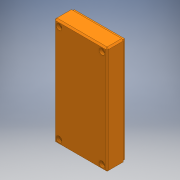
# Autodesk Inventor part: mangOH bottom
Saved by Autodesk Inventor 2017.3 (Build 213256000, 256)
## iProperties
Created: 2018-01-31
Part Number: mangOH bottom
Material: Generic
Document SubType Name: Modeling
Designer: michiel
Density: 1 g/cm^3
Appearance: Orange
Author: michiel
Autodesk Inventor part; units mm, degrees
ref_plane "YZ Plane" through (0, 0, 0) normal (1, 0, 0) x (0, 1, 0)
ref_plane "XZ Plane" through (0, 0, 0) normal (0, 1, 0) x (-1, 0, 0)
ref_plane "XY Plane" through (0, 0, 0) normal (0, 0, 1) x (1, 0, 0)
sketch "Sketch1" plane through (0, 0, 0) normal (0, 1, 0) x (-1, 0, 0)
  line L0 (0, 0) -> (73, 0)
  line L1 (73, 0) -> (73, -148)
  line L2 (73, -148) -> (0, -148)
  line L3 (0, -148) -> (0, 0)
  dimension "d0" = 73
  dimension "d1" = 148
  constraints: 8 end point, 2 parallel, 1 horizontal, 1 perpendicular
  measures "d0" distance of L1.end L2.end
  measures "d1" distance of L0.end L1.end
extrude "Extrusion1" add sketch "Sketch1" against normal blind 4
sketch "Sketch2" plane through (0, 0, 0) normal (0, 1, 0) x (1, 0, 0)
  line L0 (-73, 148) -> (0, 148) projected
  line L1 (0, 148) -> (0, 0) projected
  line L2 (0, 148) -> (0, 0)
  line L3 (0, 0) -> (-73, 0) projected
  line L4 (0, 0) -> (-73, 0)
  line L5 (-73, 0) -> (-73, 148)
  line L6 (0, 148) -> (0, 144) construction
  line L7 (0, 148) -> (0, 0) construction
  line L8 (0, 144) -> (-4, 144) construction
  line L9 (-4, 144) -> (-69, 144)
  line L10 (-69, 144) -> (-69, 4)
  line L11 (-69, 4) -> (-4, 4)
  line L12 (-4, 4) -> (-4, 144)
  dimension "d4" = 4
  dimension "d5" = 4
  dimension "d6" = 90
  dimension "d7" = 65
  dimension "d8" = 140
  constraints: 18 end point, 3 perpendicular, 2 collinear, 2 horizontal, 1 point on line, 1 vertical
  measures "d4" distance of L0.end L6.end
  measures "d5" distance of L6.end L8.end
  measures "d6" angle of L6 L8
  measures "d7" distance of L8.end L9.end
  measures "d8" distance of L9.end L10.end
extrude "Extrusion2" add sketch "Sketch2" along normal blind 22
sketch "Sketch3" plane through (0, 22, 0) normal (0, 1, 0) x (1, 0, 0)
  line L0 (-4, 4) -> (-69, 4)
  line L1 (-4, 4) -> (-2.1, 4) construction
  line L2 (-2.1, 4) -> (-2.1, 2.1) construction
  line L3 (-2.1, 2.1) -> (-71.1, 2.1)
  line L4 (-73, 148) -> (-73, 0) projected
  line L5 (-71.1, 2.1) -> (-71.1, 146.1)
  line L6 (-71.1, 146.1) -> (-2.1, 146.1)
  line L7 (-2.1, 146.1) -> (-2.1, 2.1)
  line L8 (-73, 0) -> (0, 0) projected
  line L9 (0, 148) -> (-73, 148) projected
  line L10 (-73, 0) -> (-73, 148)
  line L11 (-73, 148) -> (0, 148)
  line L12 (0, 148) -> (0, 0)
  point P0 (-4, 144)
  point P1 (-69, 144)
  dimension "d11" = 1.9
  dimension "d12" = 1.9
  dimension "d13" = 69
  dimension "d14" = 144
  dimension "d15" = 69
  constraints: 20 end point, 5 perpendicular, 2 vertical, 1 horizontal, 1 point on line
  measures "d11" distance of L0.start L1.end
  measures "d12" distance of L1.end L2.end
  measures "d13" distance of L2.end L3.end
  measures "d14" distance of L3.end L5.end
  measures "d15" distance of L5.end L6.end
extrude "Extrusion3" cut sketch "Sketch3" against normal blind 4
sketch "Sketch4" plane through (0, 0, 0) normal (0, 1, 0) x (1, 0, 0)
  line L0 (-69, 4) -> (-69, 144) projected
  line L1 (-69, 144) -> (-63, 144)
  line L2 (-63, 144) -> (-63, 138)
  line L3 (-63, 138) -> (-69, 138)
  line L4 (-69, 138) -> (-69, 144)
  point P0 (0, 0)
  dimension "d18" = 6
  dimension "d19" = 6
  constraints: 8 end point, 2 parallel, 1 horizontal, 1 perpendicular
  measures "d18" distance of L2.end L3.end
  measures "d19" distance of L1.end L2.end
extrude "Extrusion4" add sketch "Sketch4" along normal blind 15
sketch "Sketch5" plane through (0, 22, 0) normal (0, 1, 0) x (1, 0, 0)
  line L0 (-69, 138) -> (-63, 138) construction
  line L1 (-63, 138) -> (-66, 138) construction
  line L2 (-63, 138) -> (-60, 138) construction
  line L3 (-66, 138) -> (-66, 141) construction
  circle A0 centre (-66, 141) radius 2
  point P0 (0, 0)
  dimension "d22" = 3
  dimension "d23" = 180
  dimension "d24" = 3
  dimension "d25" = 4
  constraints: 6 end point, 2 collinear, 1 centre point, 1 coincident, 1 horizontal, 1 vertical
  measures "d22" distance of L0.end L1.end
  measures "d23" angle of L1 L2
  measures "d24" distance of L1.end L3.end
  measures "d25" diameter of A0
extrude "Extrusion5" cut sketch "Sketch5" against normal blind 20
sketch "Sketch6" plane through (0, -4, 0) normal (0, -1, 0) x (1, 0, 0)
  line L0 (-73, 0) -> (-73, -148) construction
  line L1 (-73, -148) -> (-73, -141) construction
  line L2 (-73, -141) -> (-66, -141) construction
  circle A0 centre (-66, -141) radius 4
  point P0 (0, 0)
  dimension "d28" = 7
  dimension "d41" = 7
  dimension "d42" = 8
  constraints: 4 end point, 1 centre point, 1 coincident, 1 horizontal, 1 point on line
  measures "d28" distance of L0.end L1.end
  measures "d41" distance of L1.end L2.end
  measures "d42" diameter of A0
extrude "Extrusion6" cut sketch "Sketch6" against normal blind 4
pattern_linear "Rectangular Pattern1" count 2 spacing 59 along (1, 0, 0) count 2 spacing 134 along (0, 0, 1) of "Extrusion4", "Extrusion5", "Extrusion6"
sketch "Sketch7" plane through (0, 0, 0) normal (0, 1, 0) x (1, 0, 0)
  line L0 (-69, 138) -> (-63, 138) projected
  line L1 (-69, 138) -> (-63, 138)
  line L2 (-10, 144) -> (-63, 144) projected
  line L3 (-63, 138) -> (-63, 144)
  line L4 (-63, 144) -> (-61.4, 144)
  line L5 (-69, 138) -> (-69, 136.4)
  line L6 (-69, 138) -> (-69, 10) projected
  line L7 (-69, 136.4) -> (-61.4, 136.4)
  line L8 (-61.4, 136.4) -> (-61.4, 144)
  point P0 (0, 0)
  dimension "d43" = 1.6
  dimension "d44" = 1.6
  constraints: 12 end point, 4 perpendicular, 1 horizontal, 1 point on line
  measures "d43" distance of L2.end L4.end
  measures "d44" distance of L0.start L5.end
extrude "Extrusion7" add sketch "Sketch7" along normal blind 1.2
sketch "Sketch8" plane through (0, 0, 0) normal (0, 1, 0) x (1, 0, 0)
  line L0 (-10, 4) -> (-10, 4.3542) projected
  line L1 (-10, 4) -> (-11.6, 4)
  line L2 (-4, 4) -> (-69, 4) projected
  line L3 (-4, 10) -> (-10, 10) projected
  line L4 (-10, 4) -> (-10, 10)
  line L5 (-10, 10) -> (-4, 10)
  line L6 (-4, 10) -> (-4, 11.6)
  line L7 (-4, 11.6) -> (-11.6, 11.6)
  line L8 (-11.6, 11.6) -> (-11.6, 4)
  line L9 (-11.6, 11.6) -> (-69, 11.6) construction
  line L10 (-69, 136.4) -> (-69, 10) projected
  line L11 (-69, 10) -> (-69, 11.6)
  line L12 (-69, 10) -> (-63, 10)
  line L13 (-63, 10) -> (-63, 4)
  line L14 (-63, 4) -> (-61.4, 4)
  line L15 (-63, 4) -> (-10, 4) projected
  line L16 (-61.4, 4) -> (-61.4, 11.6)
  line L17 (-69, 11.6) -> (-61.4, 11.6)
  line L18 (-9.6458, 138) -> (-10, 138) projected
  line L19 (-4, 138) -> (-2.4, 138) construction
  line L20 (-10, 144) -> (-61.4, 144) projected
  line L21 (-10, 138) -> (-10, 144)
  line L22 (-10, 144) -> (-11.6, 144)
  line L23 (-10, 138) -> (-4, 138)
  line L24 (-4, 138) -> (-4, 136.4)
  line L25 (-4, 10) -> (-4, 138) projected
  line L26 (-4, 136.4) -> (-11.6, 136.4)
  line L27 (-11.6, 136.4) -> (-11.6, 144)
  point P0 (0, 0)
  dimension "d47" = 1.6
  dimension "d48" = 1.6
  dimension "d49" = 1.6
  dimension "d55" = 7.6
  dimension "d56" = 7.6
  dimension "d57" = 1.6
  dimension "d58" = 1.6
  dimension "d59" = 90
  constraints: 40 end point, 6 point on line, 4 perpendicular, 3 collinear, 3 horizontal, 2 vertical
  measures "d47" distance of L0.start L1.end
  measures "d48" distance of L3.start L6.end
  measures "d49" distance of L13.end L14.end
  measures "d55" distance of L7.end L1.end
  measures "d56" distance of L6.end L7.end
  measures "d57" distance of L20.start L22.end
  measures "d58" distance of L19.start L24.end
  measures "d59" angle of L24 L26
extrude "Extrusion8" add sketch "Sketch8" along normal blind 1.2
sketch "Sketch9" plane through (-69, 15, -10) normal (0, 1, 0) x (1, 0, 0)
  line L0 (6, -6) -> (6, 0) projected
  line L1 (0, -6) -> (0, 134) projected
  line L2 (6, 0) -> (0, 0)
  line L3 (0, 0) -> (0, -6)
  line L4 (0, -6) -> (6, -6)
  line L5 (6, -6) -> (6, 0)
  line L6 (65, 134) -> (65, -6) projected
  line L7 (65, 1.6) -> (65, -6)
  line L8 (65, -6) -> (57.4, -6)
  line L9 (59, 134) -> (59, 128) projected
  line L10 (65, 134) -> (59, 134)
  line L11 (59, 134) -> (59, 128)
  line L12 (59, 128) -> (65, 128)
  line L13 (65, 128) -> (65, 134)
  line L14 (65, -6) -> (59, -6) projected
  line L15 (65, -6) -> (59, -6)
  line L16 (59, -6) -> (59, 0)
  line L17 (59, 0) -> (65, 0)
  line L18 (65, 0) -> (65, -6)
  line L19 (6, 128) -> (6, 134) projected
  line L20 (0, 134) -> (6, 134) projected
  line L21 (6, 128) -> (0, 128)
  line L22 (0, 128) -> (0, 134)
  line L23 (0, 134) -> (6, 134)
  line L24 (6, 134) -> (6, 128)
  point P0 (69, -10)
  point P1 (57.4, 1.6)
  constraints: 36 end point, 8 parallel, 4 horizontal, 4 perpendicular
extrude "Extrusion9" add sketch "Sketch9" along normal blind 6
sketch "Sketch10" plane through (-66, 0, -7) normal (0, -1, 0) x (1, 0, 0)
  circle A0 centre (0, 0) radius 2.05
  circle A1 centre (59, 0) radius 2 projected
  circle A2 centre (59, 0) radius 2.05
  circle A3 centre (0, -134) radius 2 projected
  circle A4 centre (0, -134) radius 2.05
  circle A5 centre (59, -134) radius 2.05
  point P0 (66, 7)
  dimension "d64" = 4.1
  dimension "d65" = 4.1
  dimension "d66" = 4.1
  dimension "d67" = 4.1
  constraints: 4 centre point, 2 coincident
  measures "d64" diameter of A0
  measures "d65" diameter of A2
  measures "d66" diameter of A4
  measures "d67" diameter of A5
extrude "Extrusion10" cut sketch "Sketch10" against normal blind 200 contours A0 | A1 | A3 | A5
sketch "Sketch11" plane through (-7, 0, -7) normal (0, -1, 0) x (1, 0, 0)
  circle A0 centre (0, 0) radius 2.05
  point P0 (7, 7)
  dimension "d70" = 4.1
  constraints: 1 centre point
  measures "d70" diameter of A0
extrude "Extrusion11" cut sketch "Sketch11" against normal blind 100
sketch "Sketch12" plane through (-66, 0, -141) normal (0, -1, 0) x (1, 0, 0)
  circle A0 centre (0, 0) radius 2.05
  point P0 (66, 141)
  dimension "d73" = 4.1
  constraints: 1 centre point
  measures "d73" diameter of A0
extrude "Extrusion12" cut sketch "Sketch12" against normal blind 100
chamfer "Chamfer1" distance 2 angle 45 8 edges at (-36.5, -4, 0) (-73, 7, 0) (-73, -4, -74) (0, 7, 0) (0, -4, -74) (0, 7, -148) (-36.5, -4, -148) (-73, 7, -148)
body "Solid1"
